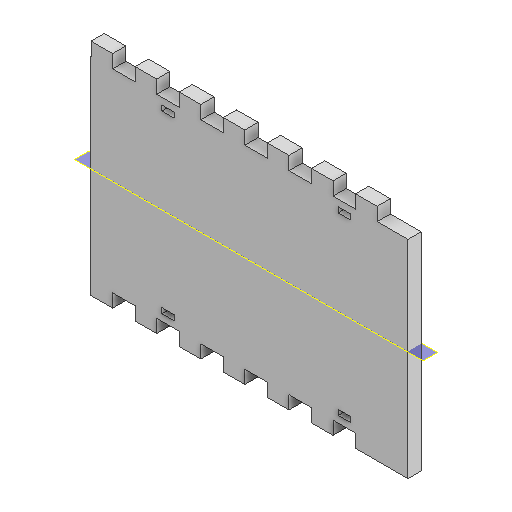
# Autodesk Inventor part: 00_Baseplate_Simmo_side7_v2
Saved by Autodesk Inventor 2022.5 (Build 265521000, 521)
## iProperties
Created: 2022-08-09
Part Number: 00_Baseplate_Simmo_side7_v2
Material: Generic
Document SubType Name: Modeling
Designer: wanghaoran
Density: 1 g/cm^3
Appearance: Default
Author: wanghaoran
Autodesk Inventor part; units mm, degrees
ref_plane "YZ Plane" through (0, 0, 0) normal (1, 0, 0) x (0, 1, 0)
ref_plane "XZ Plane" through (0, 0, 0) normal (0, 1, 0) x (-1, 0, 0)
ref_plane "XY Plane" through (0, 0, 0) normal (0, 0, 1) x (1, 0, 0)
sketch "Sketch1" plane through (0, 0, 0) normal (0, 0, 1) x (1, 0, 0)
  line L0 (-5, 11) -> (-5, 17)
  line L1 (138.883562, 11) -> (138.883562, 17)
  line L2 (138.883562, 17) -> (-5, 17)
  line L3 (-5, 17) -> (-5, -83)
  line L4 (-5, -83) -> (138.883562, -83)
  line L5 (138.883562, -83) -> (138.883562, 17)
  point P0 (0, 0)
  point P1 (-5, 17)
  dimension "d0" = 100
  constraints: 8 end point, 2 parallel, 1 horizontal, 1 perpendicular
  measures "d0" distance of L3.end L2.end
extrude "Extrusion1" add sketch "Sketch1" along normal blind 6
sketch "Sketch4" plane through (0, 0, 6) normal (0, 0, 1) x (1, 0, 0)
  line L0 (125, 6) -> (138.883562, 6)
  line L1 (125, 17) -> (125, 11)
  line L2 (138.883562, 11) -> (138.883562, 17)
  line L3 (125, 14) -> (138.883562, 14)
  line L4 (125, 11) -> (124.9, 11)
  line L5 (124.9, 11) -> (124.9, 17)
  line L6 (124.9, 17) -> (125, 17)
  line L7 (125, 17) -> (125, 11)
  point P0 (0, 0)
  dimension "d21" = 0.1
  dimension "d22" = 6
  constraints: 8 end point, 2 horizontal alignment, 2 parallel, 1 horizontal, 1 perpendicular
  measures "d21" distance of L5.end L6.end
  measures "d22" distance of L4.end L5.end
sketch "Sketch4 outline for Extrusion4" plane through (0, 0, 6) normal (0, 0, 1) x (1, 0, 0)
  line L0 (138.883562, 17) -> (124.9, 17)
  line L1 (124.9, 17) -> (124.9, 11)
  line L2 (124.9, 11) -> (138.883562, 11)
  line L3 (138.883562, 11) -> (138.883562, 17)
extrude "Extrusion4" cut sketch "Sketch4 outline for Extrusion4" against normal through all
sketch "Sketch5" plane through (0, 0, 6) normal (0, 0, 1) x (1, 0, 0)
  line L0 (115, 11) -> (115, 17) projected
  line L1 (115, 11) -> (115, 17) projected
  line L2 (105, 17) -> (115, 17) projected
  line L3 (105, 17) -> (105, 11) projected
  line L4 (105, 11) -> (115, 11) projected
  line L5 (115, 11) -> (115.1, 11)
  line L6 (115.1, 11) -> (115.1, 17)
  line L7 (115.1, 17) -> (115, 17)
  line L8 (115, 17) -> (115, 11)
  line L9 (105, 11) -> (104.9, 11)
  line L10 (104.9, 11) -> (104.9, 17)
  line L11 (104.9, 17) -> (105, 17)
  line L12 (105, 17) -> (105, 11)
  point P0 (0, 0)
  dimension "d23" = 0.1
  dimension "d24" = 6
  dimension "d25" = 0.1
  dimension "d26" = 6
  constraints: 16 end point, 4 parallel, 2 horizontal, 2 perpendicular
  measures "d23" distance of L7.end L6.end
  measures "d24" distance of L6.end L5.end
  measures "d25" distance of L10.end L11.end
  measures "d26" distance of L9.end L10.end
extrude "Extrusion5" cut sketch "Sketch5" against normal through all
pattern_linear "Rectangular Pattern2" count 6 spacing 20 along (-1, 0, 0) of "Extrusion5"
sketch "Sketch7" plane through (0, 0, 6) normal (0, 0, 1) x (1, 0, 0)
  line L0 (138.883562, 17) -> (-5, 17)
  line L1 (-5, 17) -> (-4.9, 17)
  line L2 (-4.9, 17) -> (-4.9, 11)
  line L3 (-4.9, 11) -> (-5, 11)
  line L4 (-5, 11) -> (-5, 17)
  point P0 (0, 0)
  point P1 (4.9, 17)
  point P2 (-4.9, 7.979798)
  dimension "d27" = 0.1
  dimension "d28" = 6
  constraints: 8 end point, 2 parallel, 1 horizontal, 1 perpendicular
  measures "d27" distance of L2.end L3.end
  measures "d28" distance of L1.end L2.end
extrude "Extrusion6" cut sketch "Sketch7" against normal through all
ref_plane "Work Plane1" through (-5, -33, 0) normal (0, -1, 0) x (1, 0, 0)
mirror "Mirror1" about plane through (-5, -33, 0) normal (0, -1, 0) of "Extrusion5", "Rectangular Pattern2"
sketch "Sketch8" plane through (0, 0, 6) normal (0, 0, 1) x (1, 0, 0)
  line L0 (112.75, 5.6) -> (107.25, 5.6)
  line L1 (107.25, 5.6) -> (107.25, 8)
  line L2 (107.25, 8) -> (112.75, 8)
  line L3 (112.75, 8) -> (112.75, 5.6)
  line L4 (104.9, 11) -> (104.9, 17) projected
  line L5 (115.1, 11) -> (104.9, 11) projected
  point P0 (0, 0)
  dimension "d31" = 5.5
  dimension "d32" = 2.4
  dimension "d33" = 2.35
  dimension "d34" = 3
  constraints: 8 end point, 2 parallel, 1 horizontal, 1 perpendicular
  measures "d31" distance of L1.end L2.end
  measures "d32" distance of L0.end L1.end
  measures "d33" distance between parallel lines of L4 L1
  measures "d34" distance between parallel lines of L5 L2
extrude "Extrusion7" cut sketch "Sketch8" against normal through all
pattern_linear "Rectangular Pattern3" count 2 spacing 80 along (-1, 0, 0) of "Extrusion7"
ref_plane "Work Plane2" through (138.883562, -33, 0) normal (0, -1, 0) x (1, 0, 0)
mirror "Mirror2" about plane through (138.883562, -33, 0) normal (0, -1, 0) of "Extrusion7", "Rectangular Pattern3"
body "Solid1"
